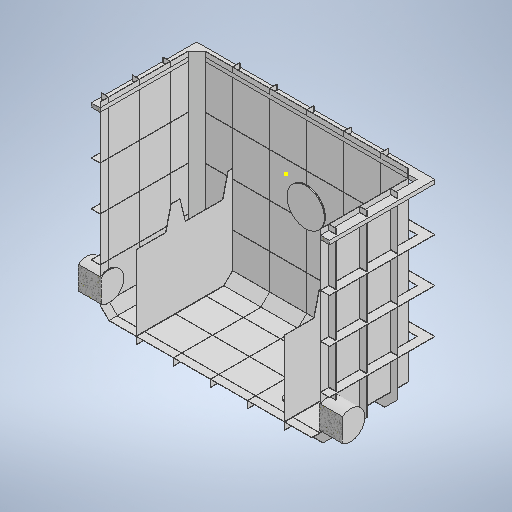
# Autodesk Inventor part: GBK-RK-0002 RK dummy
Saved by Autodesk Inventor 2026.2 (Build 302298000, 298)
## iProperties
Created: 2026-08-26
Part Number: GBK-RK-0002 RK dummy
Material: Stainless Steel
Document SubType Name: Modeling
Designer: admin
Density: 8 g/cm^3
Appearance: Default
Author: admin
Autodesk Inventor part; units mm, degrees
ref_plane "YZ Plane" through (0, 0, 0) normal (1, 0, 0) x (0, 1, 0)
ref_plane "XZ Plane" through (0, 0, 0) normal (0, 1, 0) x (-1, 0, 0)
ref_plane "XY Plane" through (0, 0, 0) normal (0, 0, 1) x (1, 0, 0)
sketch "Sketch1" plane through (0, 0, 0) normal (0, 1, 0) x (-1, 0, 0)
  line L0 (1250, 650) -> (-1250, 650)
  line L1 (-1250, 650) -> (-1250, -650)
  line L2 (-1250, -650) -> (1250, -650)
  line L3 (1250, -650) -> (1250, 650)
  line L4 (1250, 650) -> (-1250, -650) construction
  line L5 (-1250, 650) -> (1250, -650) construction
  point P0 (0, 0)
  dimension "d0" = 2500
  dimension "d1" = 1300
  constraints: 12 end point, 2 midpoint, 2 parallel, 1 horizontal, 1 perpendicular
  measures "d0" distance of L2.end L1.end
  measures "d1" distance of L1.end L0.end
extrude "Extrusion1" add sketch "Sketch1" along normal blind 100 and the other way blind 2000
chamfer "Chamfer1" distance 100 angle 45 8 edges at (0, -2000, 650) (1250, -2000, 0) (0, -2000, -650) (-1250, -2000, 0) (-1250, -950, 650) (-1250, -950, -650) (1250, -950, -650) (1250, -950, 650)
shell "Shell1" thickness 4 removed faces 1 at (383.3333, 100, -216.6667)
sketch "Sketch4" plane through (0, 0, 0) normal (0, 0, 1) x (1, 0, 0)
  line L0 (-1250, -1900) -> (-1250, 100) projected
  line L1 (-1250, 100) -> (-1250, -1900) projected
  line L2 (-1250, -1900) -> (-1150, -2000) projected
  line L3 (-1150, -2000) -> (-1250, -1900) projected
  line L4 (1150, -2000) -> (-1150, -2000) projected
  line L5 (-1150, -2000) -> (1150, -2000) projected
  line L6 (1250, -1900) -> (1150, -2000) projected
  line L7 (1150, -2000) -> (1250, -1900) projected
  line L8 (1250, 100) -> (1250, -1900) projected
  line L9 (1250, -1900) -> (1250, 100) projected
  line L10 (-1250, 100) -> (-1330, 100)
  line L11 (-1330, 100) -> (-1330, -1933.1371)
  line L12 (-1330, -1933.1371) -> (-1183.1371, -2080)
  line L13 (-1183.1371, -2080) -> (1183.1371, -2080)
  line L14 (1183.1371, -2080) -> (1330, -1933.1371)
  line L15 (1330, -1933.1371) -> (1330, 100)
  line L16 (1330, 100) -> (1250, 100)
  line L17 (0, -2000) -> (0, -2080) construction
  line L18 (-1200, -1950) -> (-1256.5685, -2006.5685) construction
  line L19 (1200, -1950) -> (1256.5685, -2006.5685) construction
  point P0 (0, 0)
  dimension "d16" = 80
  constraints: 20 end point, 7 perpendicular, 6 midpoint, 2 equal length, 2 parallel, 1 point on line
  measures "d16" distance of L1.start L10.end
sketch "Sketch2" plane through (0, 0, 0) normal (1, 0, 0) x (0, 1, 0)
  line L0 (100, -650) -> (100, 650) construction
  line L1 (100, 650) -> (100, 730)
  line L2 (100, 730) -> (-1933.1371, 730)
  line L3 (-1933.1371, 730) -> (-2080, 583.1371)
  line L4 (-2080, 583.1371) -> (-2080, -583.1371)
  line L5 (-2080, -583.1371) -> (-1933.1371, -730)
  line L6 (-1933.1371, -730) -> (100, -730)
  line L7 (100, -730) -> (100, -650)
  line L8 (-1950, -600) -> (-2006.5685, -656.5685) construction
  line L9 (-2000, 0) -> (-2080, 0) construction
  line L10 (-1950, 600) -> (-2006.5685, 656.5685) construction
  line L11 (-1900, -650) -> (-2000, -550)
  line L12 (-2000, -550) -> (-1900, -650) projected
  line L13 (-1900, 650) -> (-2000, 550)
  line L14 (-2000, 550) -> (-1900, 650) projected
  line L15 (-1900, 650) -> (100, 650)
  line L16 (100, 650) -> (-1900, 650) projected
  line L17 (100, -650) -> (-1900, -650)
  line L18 (-1900, -650) -> (100, -650) projected
  line L19 (-2000, -550) -> (-2000, 550) projected
  line L20 (-2000, 550) -> (-2000, -550) projected
  point P0 (0, 0)
  dimension "d10" = 80
  constraints: 30 end point, 6 midpoint, 6 perpendicular, 4 equal length, 2 parallel, 2 point on line
  measures "d10" distance of L0.end L1.end
extrude "Extrusion4" add sketch "Sketch4" along normal mid plane 4
extrude "Extrusion5" add sketch "Sketch2" along normal mid plane 4
pattern_linear "Rectangular Pattern2" count 5 spacing 420 along (1, 0, 0) of "Extrusion5" first direction both ways yes
pattern_linear "Rectangular Pattern3" count 3 spacing 350 along (0, 0, 1) of "Extrusion4" first direction both ways yes
sketch "Sketch5" plane through (0, 0, 0) normal (0, 1, 0) x (-1, 0, 0)
  line L0 (-1246, -548.3431) -> (-1246, 548.3431) projected
  line L1 (-1148.3431, -646) -> (-1246, -548.3431) projected
  line L2 (-1250, -650) -> (1250, -650)
  line L3 (1250, -650) -> (1250, 650)
  line L4 (1250, 650) -> (-1250, 650)
  line L5 (-1250, 650) -> (-1250, -650)
  line L6 (-1250, -650) -> (1250, 650) construction
  line L7 (1250, -650) -> (-1250, 650) construction
  line L8 (1150, 650) -> (842, 650) projected
  line L9 (1250, 352) -> (1250, 550) projected
  line L10 (-1350, -750) -> (1350, -750)
  line L11 (1350, -750) -> (1350, 750)
  line L12 (1350, 750) -> (-1350, 750)
  line L13 (-1350, 750) -> (-1350, -750)
  point P0 (0, 0)
  dimension "d29" = 100
  constraints: 20 end point, 4 parallel, 2 collinear, 2 midpoint, 2 perpendicular, 1 horizontal, 3 other
  measures "d29" distance between parallel lines of L5 L13
extrude "Extrusion6" add sketch "Sketch5" along normal blind 40
extrude "Extrusion7" add sketch "Sketch5" against normal blind 4
pattern_linear "Rectangular Pattern4" count 4 spacing 500 along (0, -1, 0) of "Extrusion7"
sketch "Sketch6" plane through (-838, -4, 730) normal (1, 0, 0) x (0, 0, -1)
  line L0 (84, -1894.3431) -> (84, 104) projected
  line L1 (84, 104) -> (84, -1894.3431) projected
  line L2 (1376, 104) -> (1376, -1894.3431) projected
  line L3 (1376, -1894.3431) -> (1376, 104) projected
  line L4 (1375.6145, -1894.7287) -> (1278.7287, -1991.6145) projected
  line L5 (1375.6145, -1894.7287) -> (1376, -1894.3431) projected
  line L6 (1376, -1894.3431) -> (1375.6145, -1894.7287) projected
  line L7 (1278.7287, -1991.6145) -> (1375.6145, -1894.7287) projected
  line L8 (1278.7287, -1991.6145) -> (1278.3431, -1992) projected
  line L9 (1278.3431, -1992) -> (1278.7287, -1991.6145) projected
  line L10 (1278.3431, -1992) -> (181.6569, -1992) projected
  line L11 (181.6569, -1992) -> (1278.3431, -1992) projected
  line L12 (84.3855, -1894.7287) -> (181.2713, -1991.6145) projected
  line L13 (84.3855, -1894.7287) -> (84, -1894.3431) projected
  line L14 (84, -1894.3431) -> (84.3855, -1894.7287) projected
  line L15 (181.2713, -1991.6145) -> (84.3855, -1894.7287) projected
  line L16 (181.6569, -1992) -> (181.2713, -1991.6145) projected
  line L17 (181.6569, -1992) -> (181.2713, -1991.6145) projected
  line L18 (84, -892) -> (730, -892)
  line L19 (134, -892) -> (194.5, -1142)
  line L20 (194.5, -1142) -> (619.5, -1142)
  line L21 (619.5, -1142) -> (680, -892)
  line L22 (730, -892) -> (730, -1992) construction
  line L23 (730, -892) -> (1376, -892)
  line L24 (407, -1142) -> (407, -892) construction
  line L25 (1326, -892) -> (1265.5, -1142)
  line L26 (1265.5, -1142) -> (840.5, -1142)
  line L27 (840.5, -1142) -> (780, -892)
  point P0 (730, 4)
  point P1 (84, -892)
  point P2 (1376, -892)
  point P3 (1326, -892)
  point P4 (780, -892)
  dimension "d37" = 425
  dimension "d38" = 1100
  dimension "d39" = 50
  dimension "d40" = 850
  constraints: 20 end point, 4 point on line, 4 symmetric about line, 3 midpoint, 2 perpendicular, 2 vertical, 1 equal length, 1 horizontal, 1 other
  measures "d37" distance of L19.end L20.end
  measures "d38" distance between parallel lines of L10 L18
  measures "d39" distance of L18.start L19.start
  measures "d40" distance between parallel lines of L10 L20
extrude "Extrusion8" add sketch "Sketch6" against normal blind 4 contours L0 L18 L19 L20 L21 L23 L27 L26 L25 L2 L5 L4 L8 L10 L16 L12 L13
mirror "Mirror1" about plane through (0, 0, 0) normal (1, 0, 0) of "Extrusion8"
sketch "Sketch7" plane through (838, -1146, 110.5) normal (-1, 0, 0) x (0, 0, 1)
  line L0 (-646, 0) -> (-706.5, 250) projected
  line L1 (-221, 0) -> (-646, 0) projected
  line L2 (-160.5, 250) -> (-221, 0) projected
  line L3 (-706.5, 250) -> (-756.5, 250) projected
  line L4 (-706.5, 250) -> (-160.5, 250)
  point P0 (-110.5, 1146)
  constraints: 2 end point, 1 horizontal
extrude "Extrusion9" add sketch "Sketch7" against normal blind 4
sketch "Sketch8" plane through (-1246, -1898.3431, -548.3431) normal (1, 0, 0) x (0, 0, -1)
  line L0 (0, 0) -> (0, 1998.3431) projected
  line L1 (-1096.6863, 1998.3431) -> (0, 1998.3431) projected
  line L2 (-1096.6863, 1998.3431) -> (-1096.6863, 0) projected
  line L3 (-1096.6863, 0) -> (0, 0) projected
  circle A0 centre (-898.3431, 148.3431) radius 162.5
  point P0 (-548.3431, 1898.3431)
  point P1 (-548.3431, 0)
  dimension "d45" = 325
  dimension "d46" = 350
  dimension "d47" = 1850
  constraints: 1 centre point, 1 midpoint
  measures "d45" diameter of A0
  measures "d46" horizontal distance of point (-548.343, 0) A0.centre
  measures "d47" distance from line of A0.centre L1
sketch "Sketch9" plane through (418, -4, 650) normal (-1, 0, 0) x (0, 0, 1)
  point P0 (-650, 4)
sketch "Sketch10" plane through (-838, -1996, 548.3431) normal (0, 1, 0) x (1, 0, 0)
  line L0 (1676, 0) -> (1676, 1096.6863) projected
  line L1 (1676, 1096.6863) -> (0, 1096.6863) projected
  line L2 (0, 1096.6863) -> (0, 0) projected
  line L3 (0, 0) -> (1676, 0) projected
  circle A0 centre (1476, 350) radius 50
  point P0 (838, 548.3431)
  dimension "d48" = 100
  dimension "d49" = 200
  dimension "d50" = 350
  constraints: 1 centre point
  measures "d48" diameter of A0
  measures "d49" distance from line of A0.centre L0
  measures "d50" distance from line of A0.centre L3
extrude "Extrusion10" add sketch "Sketch10" along normal blind 10 and the other way blind 200 contours A0
extrude "Extrusion11" add sketch "Sketch8" along normal blind 10 and the other way blind 250 contours A0 L3 | L3 A0
mirror "Mirror2" about plane through (0, 0, 0) normal (1, 0, 0) of "Extrusion11"
mirror "Mirror3" about plane through (0, 0, 0) normal (0, 0, 1) of "Extrusion11"
sketch "Sketch11" plane through (-1148.3431, 100, -646) normal (0, 0, 1) x (1, 0, 0)
  line L0 (1990.3431, -996) -> (1990.3431, -1998.3431) projected
  line L1 (1990.3431, -1998.3431) -> (2296.6863, -1998.3431) projected
  line L2 (2296.6863, -1998.3431) -> (2296.6863, 0) projected
  line L3 (0, 0) -> (2296.6863, 0) projected
  line L4 (0, 0) -> (0, -1998.3431) projected
  line L5 (0, -1998.3431) -> (306.3431, -1998.3431) projected
  line L6 (306.3431, -1998.3431) -> (306.3431, -996) projected
  line L7 (306.3431, -996) -> (310.3431, -996) projected
  line L8 (310.3431, -996) -> (310.3431, -1998.3431) projected
  line L9 (310.3431, -1998.3431) -> (1986.3431, -1998.3431) projected
  line L10 (1986.3431, -1998.3431) -> (1986.3431, -996) projected
  line L11 (1986.3431, -996) -> (1990.3431, -996) projected
  circle A0 centre (1148.3431, -950) radius 213
  point P0 (1148.3431, -100)
  point P1 (1148.3431, 0)
  dimension "d59" = 426
  dimension "d60" = 950
  constraints: 1 centre point, 1 midpoint, 1 vertical alignment
  measures "d59" diameter of A0
  measures "d60" distance from line of L3 A0.centre
extrude "Extrusion12" add sketch "Sketch11" along normal blind 10 and the other way blind 250 contours A0
body "Solid1"
